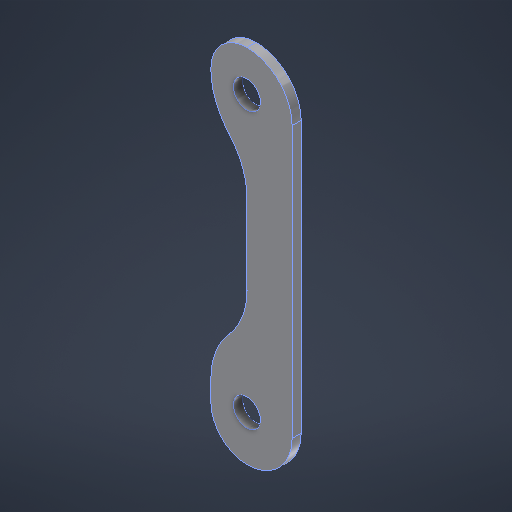
# Autodesk Inventor part: arm1
Saved by Autodesk Inventor 2025.3 (Build 293356000, 356)
## iProperties
Created: 2016-01-09
Part Number: arm1
Material: ABS Plastic
Document SubType Name: Modeling
Designer: Nanjar
Density: 1.06 g/cm^3
Appearance: Aluminum - Flat
Author: Nanjar
Autodesk Inventor part; units mm, degrees
ref_plane "YZ Plane" through (0, 0, 0) normal (1, 0, 0) x (0, 1, 0)
ref_plane "XZ Plane" through (0, 0, 0) normal (0, 1, 0) x (-1, 0, 0)
ref_plane "XY Plane" through (0, 0, 0) normal (0, 0, 1) x (1, 0, 0)
sketch "Sketch1" plane through (0, 0, 0) normal (0, 0, 1) x (1, 0, 0)
  circle A0 centre (0, 0) radius 1.5
  circle A1 centre (0, 30.5) radius 1.5
  line L0 (0, 8.5) -> (-4, 4.5)
  line L1 (-4, 35) -> (-4, 25.5)
  line L2 (-4, 4.5) -> (-4, -5)
  line L3 (0, 21) -> (0, 8.5)
  line L4 (-4, 35) -> (5, 35)
  line L5 (-4, -5) -> (5, -5)
  line L6 (5, 35) -> (5, -5)
  line L7 (0, 21) -> (0, 23.5)
  line L8 (-4, 25.5) -> (-4, 28)
  line L9 (-4, 28) -> (0, 23.5)
  dimension "d0" = 3
  dimension "d1" = 3
  dimension "d47" = 9
  dimension "d48" = 9
  dimension "d52" = 4
  dimension "d55" = 4.5
  dimension "d59" = 40
  dimension "d60" = 2.5
  dimension "d61" = 2.5
  constraints: 20 end point, 4 vertical, 2 centre point, 2 horizontal, 1 coincident, 1 collinear, 1 point on line
  measures "d0" diameter of A0
  measures "d1" diameter of A1
  measures "d47" distance of L1.start L4.end
  measures "d48" distance of L2.end L5.end
  measures "d52" distance from line of L1 A1.centre
  measures "d55" distance from line of L4 A1.centre
  measures "d59" distance of L4.end L5.end
  measures "d60" distance of L3.start L7.end
  measures "d61" distance of L1.end L8.end
extrude "Extrusion1" add sketch "Sketch1" along normal blind 1
fillet "Fillet9" radius 5 2 edges at (5, 35, 0.5) (5, -5, 0.5)
fillet "Fillet10" radius 4 2 edges at (-4, 35, 0.5) (-4, -5, 0.5)
fillet "Fillet11" radius 7.8 2 edges at (0, 8.5, 0.5) (-4, 4.5, 0.5)
fillet "Fillet12" radius 7.8 2 edges at (-4, 28, 0.5) (0, 23.5, 0.5)
body "Solid1"
